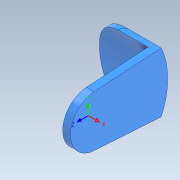
# Autodesk Inventor part: shank_connector
Saved by Autodesk Inventor 2020 (Build 240168000, 168)
## iProperties
Created: 2021-03-27
Part Number: shank_connector
Material: Generic
Document SubType Name: Modeling
Designer: DELL
Density: 1 g/cm^3
Appearance: Cyan
Author: DELL
Autodesk Inventor part; units mm, degrees
ref_plane "YZ Plane" through (0, 0, 0) normal (1, 0, 0) x (0, 1, 0)
ref_plane "XZ Plane" through (0, 0, 0) normal (0, 1, 0) x (-1, 0, 0)
ref_plane "XY Plane" through (0, 0, 0) normal (0, 0, 1) x (1, 0, 0)
sketch "Sketch1" plane through (0, 0, 0) normal (1, 0, 0) x (0, 1, 0)
  circle A0 centre (0, 0) radius 20
  line L0 (-19.9583, 1.2905) -> (-23.3333, -50.9073)
  line L1 (19.9583, 1.2905) -> (23.3333, -50.9073)
  line L2 (9.9593, -5.75) -> (0, 0) construction
  line L3 (0, -48.5721) -> (0, 22.5) construction
  arc A1 (-23.0554, -46.6095) -> (23.0554, -46.6095) centre (0, 0) ccw
  arc A2 (-23.3333, -50.9073) -> (23.3333, -50.9073) centre (0, 0) ccw
  line L4 (0, 0) -> (-23.3333, -50.9073) construction
  point P0 (0, 11.4686)
  point P1 (0, 11.4686)
  dimension "d0" = 40
  dimension "d8" = 104
  dimension "d9" = 112
  dimension "d10" = 24.624
  constraints: 10 end point, 6 point on circle, 5 coincident, 3 centre point, 3 point on line, 2 tangent, 1 vertical, 1 other
  measures "d0" diameter of A0
  measures "d8" diameter of A1
  measures "d9" diameter of A2
  measures "d10" angle of L3 L4
extrude "Extrusion1" add sketch "Sketch1" along normal blind 6
extrude "Extrusion2" add sketch "Sketch1" against normal blind 47.5 from surface at 0 contours L1 A2 L0 A1
sketch "Sketch2" plane through (0, 0, 0) normal (0, 0, 1) x (1, 0, 0)
  line L0 (6, -19.9583) -> (6, 19.9583) construction
  line L1 (6, 0) -> (-47.5, 0) construction
  line L2 (-47.5, 23.3333) -> (-47.5, -23.3333) projected
  circle A0 centre (-20, 0) radius 23.3333
  line L3 (6, 23.3333) -> (-47.5, 23.3333) projected
  line L4 (-47.5, -23.3333) -> (6, -23.3333) projected
  line L5 (-20, 23.3333) -> (-20, -23.3333) construction
  point P0 (0, 0)
  dimension "d21" = 27.5
  constraints: 4 end point, 3 point on line, 2 midpoint, 2 point on circle, 2 tangent, 1 centre point
  measures "d21" distance between parallel lines of L2 L5
extrude "Extrusion3" cut sketch "Sketch2" against normal through all contours L3 A0 L4 L2
body "Solid1"
